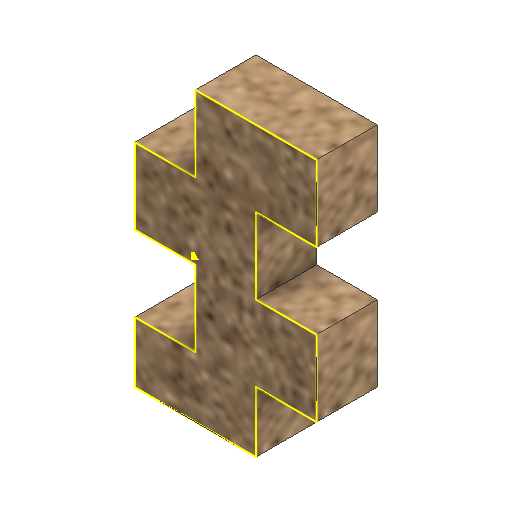
# Autodesk Inventor part: wall2
Saved by Autodesk Inventor 2025 (Build 290162000, 162)
## iProperties
Created: 2024-09-26
Part Number: wall2
Material: MDF Medium Density Fiberboard
Document SubType Name: Modeling
Designer: DANIEL
Density: 0.8 g/cm^3
Appearance: Cardboard - Corrugated
Checked By: FERNANDO
Engr Approved By: ANTONIO
Stock Number: 8
Mass: 0.4864 g
Surface Area: 6.16 cm^2
Volume: 0.608 cm^3
Author: DANIEL
Title: WALL 2
Autodesk Inventor part; units mm, degrees
ref_plane "YZ Plane" through (0, 0, 0) normal (1, 0, 0) x (0, 1, 0)
ref_plane "XZ Plane" through (0, 0, 0) normal (0, 1, 0) x (-1, 0, 0)
ref_plane "XY Plane" through (0, 0, 0) normal (0, 0, 1) x (1, 0, 0)
sketch "Sketch1" plane through (0, 0, 0) normal (0, 0, 1) x (1, 0, 0)
  line L0 (-4, 9.5) -> (4, 9.5)
  line L1 (4, 9.5) -> (4, -9.5)
  line L2 (4, -9.5) -> (-4, -9.5)
  line L3 (-4, -9.5) -> (-4, 9.5)
  line L4 (-4, 9.5) -> (4, -9.5) construction
  line L5 (4, 9.5) -> (-4, -9.5) construction
  line L6 (4, 9.5) -> (8, 9.5)
  line L7 (8, 9.5) -> (8, 4.5)
  line L8 (8, 4.5) -> (4, 4.5)
  line L9 (4, 4.5) -> (4, 9.5)
  line L10 (8, -0.5) -> (4, -0.5)
  line L11 (8, 4.5) -> (8, -0.5)
  line L12 (8, -5.5) -> (4, -5.5)
  line L13 (8, -0.5) -> (8, -5.5)
  line L14 (2, 14.112) -> (2, 5.4586)
  line L15 (0, 9.5) -> (0, -9.5)
  line L16 (0, 9.5) -> (-4, 9.5)
  line L17 (-4, 9.5) -> (-4, 4.5)
  line L18 (-4, 4.5) -> (0, 4.5)
  line L19 (-4, -0.5) -> (0, -0.5)
  line L20 (-4, 4.5) -> (-4, -0.5)
  line L21 (-4, -0.5) -> (-4, -9.5)
  line L22 (-4, -5.5) -> (0, -5.5)
  point P0 (0, 0)
  point P1 (0, 4.5)
  point P2 (-4, 4.5)
  point P3 (-4, -0.5)
  point P4 (4, -7)
  point P5 (8, -0.5)
  point P6 (0, 9.5)
  point P7 (8, 4.5)
  point P8 (4, -5.5)
  point P9 (0, -5.5)
  point P10 (-4, -5.5)
  dimension "d0" = 8
  dimension "d1" = 19
  dimension "d2" = 4
  dimension "d3" = 5
  dimension "d6" = 5
  dimension "d11" = 12
  dimension "d12" = 6
  constraints: 46 end point, 10 symmetric about line, 4 parallel, 2 horizontal, 2 midpoint, 2 perpendicular, 2 vertical, 10 other
  measures "d0" distance of L1.end L2.end
  measures "d1" distance of L0.end L1.end
  measures "d2" distance of L7.end L8.end
  measures "d3" distance of L6.end L7.end
  measures "d6" distance of L7.end L10.start
  measures "d11" distance between parallel lines of L3 L13
  measures "d12" distance between parallel lines of L7 L14
extrude "Extrusion1" add sketch "Sketch1" along normal blind 4 contours L0 L1 L2 L15 | L18 L15 L19 L3 | L6 L7 L8 L1 | L22 L15 L2 L3 | L10 L13 L12 L1
sketch "Sketch2" plane through (0, 0, 4) normal (0, 0, 1) x (1, 0, 0)
  line L0 (0, -5.5) -> (-4, -5.5) projected
  line L1 (-4, -5.5) -> (-4, -9.5) projected
  line L2 (-4, -9.5) -> (4, -9.5) projected
  line L3 (4, -9.5) -> (4, -5.5) projected
  line L4 (4, -5.5) -> (8, -5.5) projected
  line L5 (8, -5.5) -> (8, -0.5) projected
  line L6 (8, -0.5) -> (4, -0.5) projected
  line L7 (4, -0.5) -> (4, 4.5) projected
  line L8 (4, 4.5) -> (8, 4.5) projected
  line L9 (8, 4.5) -> (8, 9.5) projected
  line L10 (8, 9.5) -> (0, 9.5) projected
  line L11 (0, 9.5) -> (0, 4.5) projected
  line L12 (0, 4.5) -> (-4, 4.5) projected
  line L13 (-4, 4.5) -> (-4, -0.5) projected
  line L14 (-4, -0.5) -> (0, -0.5) projected
  line L15 (0, -0.5) -> (0, -5.5) projected
  point P0 (0, 0)
equation "\"d1\" = height + e"
equation "\"d2\" = e"
equation "\"d3\" = 0.333333 * height"
equation "\"d6\" = d3"
equation "\"d12\" = 0.5 * d11"
equation "\"d13\" = e"
equation "\"e\" = 4"
equation "\"height\" = 15"
body "Solid1"
